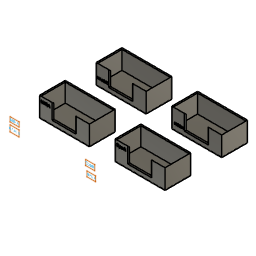
thelio-io-holder v2 (Autodesk Fusion 360 design; units mm, degrees)
Autodesk Fusion 360 part; units mm, degrees
sketch "Sketch1" plane through (0, 0, 0) normal (0, 0, 1) x (1, 0, 0)
  line L0 (-200, 150) -> (-134, 150)
  line L1 (-134, 150) -> (-134, 116)
  line L2 (-134, 116) -> (-200, 116)
  line L3 (-200, 116) -> (-200, 150)
  dimension "d1" = 66
  dimension "d2" = 34
  constraint horizontal L0
  constraint vertical L1
  constraint horizontal L2
  constraint vertical L3
  measures "d1" distance of L0.start L0.end
  measures "d2" distance of L0.start L2.end
extrude "Extrude1" add sketch "Sketch1" along normal blind 26 makes body 1
shell "Shell1" thickness 1 removed faces 1 at (-178, 138.6667, 26) on bodies 1
sketch "Sketch2" plane through (0, 116, 0) normal (0, -1, 0) x (1, 0, 0)
  line L0 (-200, 0) -> (-134, 0)
  line L1 (-134, 0) -> (-134, 26)
  line L2 (-134, 26) -> (-200, 26)
  line L3 (-200, 26) -> (-200, 0)
  line L4 (-182.0469, 26) -> (-182.0469, 7)
  line L5 (-182.0469, 7) -> (-153, 7)
  line L6 (-153, 7) -> (-153, 26)
  constraint coincident L2 L4.start
  constraint perpendicular L2 L4
  constraint perpendicular L4 L5
  constraint coincident L2 L6.end
  constraint perpendicular L2 L6
extrude "Extrude2" cut sketch "Sketch2" against normal blind 3 contours L2 L4 L5 L6 bodies 1
fillet "Fillet1" radius 1.5 3 edges at (-182.0469, 116, 16.5) (-167.5235, 116, 7) (-153, 116, 16.5) on bodies 1
fillet "Fillet2" radius 1 5 edges at (-199, 133, 26) (-167, 149, 26) (-135, 133, 26) (-144, 117, 26) (-190.5235, 117, 26) on bodies 1
copy_body "CopyPasteBodies1" bodies 1 makes body 2
move_body "Move1" bodies 2 to x (1, 0, 0) y (0, 1, 0) z (0, 0, 1) at (-100, 0, 0)
copy_body "CopyPasteBodies2" bodies 1 makes body 3
move_body "Move2" bodies 3 to x (1, 0, 0) y (0, 1, 0) z (0, 0, 1) at (0, -75, 0)
copy_body "CopyPasteBodies3" bodies 1 makes body 4
move_body "Move3" bodies 4 to x (1, 0, 0) y (0, 1, 0) z (0, 0, 1) at (-100, -75, 0)
sketch "Sketch3" plane through (0, 0, 0) normal (0, 1, 0) x (1, 0, 0)
  line L0 (-298, -17) -> (-286, -17) construction
  line L1 (-286, -17) -> (-286, -23) construction
  line L2 (-286, -23) -> (-298, -23) construction
  line L3 (-298, -23) -> (-298, -17) construction
  line L4 (-198, -17) -> (-186, -17) construction
  line L5 (-186, -17) -> (-186, -24) construction
  line L6 (-186, -24) -> (-198, -24) construction
  line L7 (-198, -24) -> (-198, -17) construction
  line L8 (-298.0132, -5.6074) -> (-286.1146, -5.6074) construction
  line L9 (-286.1146, -5.6074) -> (-286.1146, -13.6766) construction
  line L10 (-286.1146, -13.6766) -> (-298.0132, -13.6766) construction
  line L11 (-298.0132, -13.6766) -> (-298.0132, -5.6074) construction
  line L12 (-196.2552, -5) -> (-185, -5) construction
  line L13 (-185, -5) -> (-185, -11.6503) construction
  line L14 (-185, -11.6503) -> (-196.2552, -11.6503) construction
  line L15 (-196.2552, -11.6503) -> (-196.2552, -5) construction
  dimension "d12" = 3.5
  dimension "d13" = 3.5
  dimension "d16" = 3
  dimension "d17" = 3
  text T0 "MIRA" font "Arial" height 3.5 align centre middle in box 12 x 6 at (-298, -17) x (1, 0) y (0, -1) spacing 1
  text T1 "Spark" font "Arial" height 3.5 align centre middle in box 12 x 7 at (-198, -17) x (1, 0) y (0, -1) spacing 1
  text T2 "MAJOR" font "Arial" height 3 align centre middle in box 11.8986 x 8.0692 at (-298.0132, -5.6074) x (1, 0) y (0, -1) spacing 1
  text T3 "MEGA" font "Arial" height 3 align centre middle in box 11.2552 x 6.6503 at (-196.2552, -5) x (1, 0) y (0, -1) spacing 1
extrude "Extrude3" cut sketch "Sketch3" along normal blind 0.2 from surface at 41 text T0 T1 bodies 3 4
extrude "Extrude4" cut sketch "Sketch3" along normal blind 0.2 from surface at 116 text T2 T3 bodies 1 2
